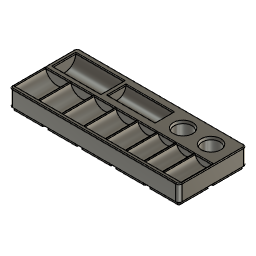
HarborFreightSocketHolder_LargeImperial (Autodesk Fusion 360 design; units mm, degrees)
Autodesk Fusion 360 part; units mm, degrees
sketch "Sketch1" plane through (0, 0, 0) normal (0, 0, 1) x (1, 0, 0) in component "Blank Storage"
  line L0 (0, 42) -> (42, 42)
  line L1 (42, 42) -> (42, 0)
  line L2 (42, 0) -> (0, 0)
  line L3 (0, 0) -> (0, 42)
  line L4 (0, 42) -> (42, 0) construction
  line L5 (42, 21) -> (0, 21) construction
  line L6 (42, 14.5) -> (0, 14.5)
  line L7 (42, 27.5) -> (0, 27.5)
  line L8 (27.5, 42) -> (27.5, 0)
  line L9 (14.5, 42) -> (14.5, 0)
  line L10 (14.5, 14.5) -> (0, 0) construction
  circle A0 centre (8, 8) radius 1.5
  circle A1 centre (34, 8) radius 1.5
  circle A2 centre (34, 34) radius 1.5
  circle A3 centre (8, 34) radius 1.5
  circle A4 centre (8, 8) radius 3.25
  circle A5 centre (34, 8) radius 3.25
  circle A6 centre (34, 34) radius 3.25
  circle A7 centre (8, 34) radius 3.25
  point P0 (21, 21)
  dimension "d1" = 42
  dimension "d2" = 42
  dimension "d65" = 13
  dimension "d67" = 90
  dimension "d69" = 3
  dimension "d71" = 360
  dimension "d80" = 6.5
  dimension "d85" = 8
  constraint horizontal L0
  constraint perpendicular L0 L1
  constraint parallel L0 L2
  constraint parallel L1 L3
  constraint coincident L2.end L3.start
  constraint midpoint L1 L5.start
  constraint midpoint L3 L5.end
  constraint coincident L1 L6.start
  constraint coincident L3 L6.end
  constraint perpendicular L3 L6
  constraint symmetric L5 L6.start L7.start
  constraint symmetric L5 L6.end L7.end
  constraint midpoint L4 P0
  constraint coincident L9 L10.start
  constraint coincident L6 L10.start
  constraint concentric A0 A4
  constraint coincident L10 A0.centre
  measures "d1" distance of L1.end L2.end
  measures "d2" distance of L0.end L1.end
  measures "d65" distance of L6 L7
  measures "d69" diameter of A0
  measures "d80" diameter of A4
  measures "d85" distance of L2 A0.centre
extrude "Extrude1" add sketch "Sketch1" along normal blind 5 contours L0 L3 L7 L9 | L0 L7 L8 L9 | L3 L6 L7 L9 | L0 L1 L7 L8 | L6 L7 L8 L9 | L2 L3 L6 L9 | L1 L6 L7 L8 | L2 L6 L8 L9 | L1 L2 L6 L8 | A0 | A1 | A2 | A3 | A4 | A5 | A6 | A7 makes body 1 in component "Blank Storage"
ref_plane "WorkPlane1" through (21, 21, 2.5) normal (0, -1, 0) x (1, 0, 0) in component "Blank Storage"
sketch "Sketch2" plane through (0, 21, 0) normal (0, -1, 0) x (1, 0, 0) in component "Blank Storage"
  line L0 (42, 0) -> (0, 0)
  line L1 (0, 0) -> (0, 5)
  line L2 (3.2, 0) -> (2.4, 0.8)
  line L3 (3.2, 0) -> (0, 0) construction
  line L4 (2.4, 0.8) -> (2.4, 2.6)
  line L5 (2.4, 2.6) -> (0, 5)
  line L6 (0, 5) -> (-5.1222, 5)
  line L7 (-5.1222, 5) -> (-5.1222, -0.0937)
  line L8 (-5.1222, -0.0937) -> (0, 0)
  dimension "d39" = 45
  dimension "d40" = 45
  dimension "d41" = 0.8
  dimension "d43" = 5
  dimension "d112" = 2.4
  constraint horizontal L3
  constraint coincident L0 L2.start
  constraint perpendicular L0 L4
  constraint coincident L1 L5.end
  constraint coincident L0.end L1.start
  constraint coincident L1.end L5.end
  constraint perpendicular L1 L6
  constraint perpendicular L6 L7
  measures "d39" angle of L2 L3
  measures "d40" angle of L4 L5
  measures "d41" distance of L2.end L3
  measures "d43" distance of L3 L1.end
  measures "d112" horizontal distance of L0.end L2.end
sketch "Sketch3" plane through (0, 0, 0) normal (0, 0, -1) x (1, 0, 0)
  line L0 (42, 0) -> (0, 0)
  line L1 (0, 0) -> (0, -42)
  line L2 (0, -42) -> (42, -42)
  line L3 (42, -42) -> (42, 0)
  arc A0 (4, 0) -> (0, -4) centre (4, -4) ccw
  line L4 (0, -42) -> (42, 0) construction
  arc A1 (0, -38) -> (4, -42) centre (4, -38) ccw
  arc A2 (38, -42) -> (42, -38) centre (38, -38) ccw
  arc A3 (42, -4) -> (38, 0) centre (38, -4) ccw
  line L5 (0, -4) -> (0, -38)
  line L6 (4, -42) -> (38, -42)
  line L7 (42, -38) -> (42, -4)
  line L8 (38, 0) -> (4, 0)
  point P0 (21, -21)
  dimension "d37" = 360
  constraint coincident L1.end L2.start
  constraint coincident L0.start L3.end
  constraint midpoint L4 P0
sweep "Sweep1" cut profiles "Sketch2" path "Sketch3" along L8 A0 L5 A1 L6 A2 L7 A3 section 1 bodies 1 in component "Blank Storage"
extrude "Extrude3" [suppressed] in component "Blank Storage"
draft "Draft1" [suppressed] in component "Blank Storage"
extrude "Extrude4" cut sketch "Sketch1" along normal up to surface (5 mm away) contours A0 | A1 | A2 | A3 bodies 1 in component "Blank Storage"
extrude "Extrude5" cut sketch "Sketch1" along normal blind 2.4 contours A4 | A5 | A6 | A7 bodies 1 in component "Blank Storage"
chamfer "Chamfer1" distance 1.75 angle 45 4 edges at (33.4576, 6.6015, 2.4) (35.3985, 33.4576, 2.4) (8.5424, 35.3985, 2.4) (6.6015, 8.5424, 2.4) on bodies 1 in component "Blank Storage"
pattern_linear "R-Pattern1" count 5 spacing 42 along (1, 0, 0) count 2 spacing 42 along (0, 1, 0) of bodies 1 makes body 2 at (66.9668, 17.0068, 5) makes body 3 at (24.9668, 59.0068, 5) makes body 4 at (66.9668, 59.0068, 5) makes body 5 at (108.9668, 17.0068, 5) makes body 6 at (108.9668, 59.0068, 5) makes body 7 at (150.9668, 17.0068, 5) makes body 8 at (192.9668, 17.0068, 5) makes body 9 at (150.9668, 59.0068, 5) makes body 10 at (192.9668, 59.0068, 5) in component "Blank Storage"
sketch "Sketch4" plane through (0, 0, 5) normal (0, 0, 1) x (-1, 0, 0) in component "Blank Storage"
  line L0 (-4, 0) -> (-206, 0)
  line L1 (-210, -4) -> (-210, -80)
  line L2 (-206, -84) -> (-4, -84)
  line L3 (0, -80) -> (0, -4)
  arc A0 (0, -4) -> (-4, 0) centre (-4, -4) ccw
  arc A1 (-206, 0) -> (-210, -4) centre (-206, -4) ccw
  arc A2 (-210, -80) -> (-206, -84) centre (-206, -80) ccw
  arc A3 (-4, -84) -> (0, -80) centre (-4, -80) ccw
  line L4 (-206, -83.75) -> (-4, -83.75)
  arc A4 (-4, -83.75) -> (-0.25, -80) centre (-4, -80) ccw
  line L5 (-0.25, -80) -> (-0.25, -4)
  arc A5 (-0.25, -4) -> (-4, -0.25) centre (-4, -4) ccw
  line L6 (-4, -0.25) -> (-206, -0.25)
  arc A6 (-206, -0.25) -> (-209.75, -4) centre (-206, -4) ccw
  line L7 (-209.75, -4) -> (-209.75, -80)
  arc A7 (-209.75, -80) -> (-206, -83.75) centre (-206, -80) ccw
  point P0 (-210, 0)
  point P1 (0, -84)
  dimension "d44" = 210
  dimension "d45" = 84
  dimension "d48" = 4
  dimension "d49" = 4
  dimension "d50" = 4
  dimension "d51" = 4
  dimension "d118" = -0.25
  constraint horizontal L0
  constraint vertical L1
  constraint horizontal L2
  constraint vertical L3
  constraint coincident origin L0
  constraint coincident origin L3
  constraint tangent L0 A0
  constraint tangent L3 A0
  constraint coincident P0 L0
  constraint coincident P0 L1
  constraint tangent L0 A1
  constraint tangent L1 A1
  constraint tangent L1 A2
  constraint tangent L2 A2
  constraint coincident P1 L2
  constraint coincident P1 L3
  constraint tangent L2 A3
  constraint tangent L3 A3
  measures "d44" distance of origin P0
  measures "d45" distance of origin P1
  measures "d48" radius of A0
  measures "d49" radius of A1
  measures "d50" radius of A2
  measures "d51" radius of A3
extrude "Extrude2" add sketch "Sketch4" along normal blind 20 contours L0 L1 L2 L3 A0 A1 A2 A3 | L4 A4 L5 A5 L6 A6 L7 A7 bodies 1 5 6 3 4 2 in component "Blank Storage"
ref_plane "WorkPlane2" through (105, 5, 15) normal (0, -1, 0) x (1, 0, 0)
sketch "Sketch7" plane through (105, 5, 15) normal (0, -1, 0) x (1, 0, 0)
  circle A0 centre (-88.4, 13) radius 15
  circle A1 centre (-58.4, 13) radius 14
  line L0 (-88.4, 13) -> (92.4, 13) construction
  circle A2 centre (-30.4, 13) radius 13
  circle A3 centre (22.5, 13) radius 11.9
  circle A4 centre (46.4, 13) radius 11
  circle A5 centre (69.4, 13) radius 11
  circle A6 centre (92.4, 13) radius 11
  circle A7 centre (-3.4, 13) radius 13
  line L1 (-101, 10) -> (101, 10)
  line L2 (-105, -10) -> (-105, 10)
  line L3 (105, -10) -> (105, 10)
  point P0 (-103.4, 13)
  point P1 (103.4, 13)
  point P2 (-73.4, 13)
  point P3 (-72.4, 13)
  point P4 (-44.4, 13)
  point P5 (-43.4, 13)
  point P6 (-17.4, 13)
  point P7 (-16.4, 13)
  point P8 (9.6, 13)
  point P9 (10.6, 13)
  point P10 (34.4, 13)
  point P11 (35.4, 13)
  point P12 (57.4, 13)
  point P13 (58.4, 13)
  point P14 (80.4, 13)
  point P15 (81.4, 13)
  dimension "d194" = 30
  dimension "d195" = 28
  dimension "d196" = 26
  dimension "d197" = 23.8
  dimension "d198" = 22
  dimension "d199" = 22
  dimension "d200" = 22
  dimension "d201" = 26
  dimension "d232" = 3
  dimension "d236" = 1
  dimension "d237" = 1
  dimension "d238" = 1
  dimension "d239" = 1
  dimension "d240" = 1
  dimension "d241" = 1
  dimension "d242" = 1
  dimension "d243" = 1.6
  dimension "d244" = 1.6
  constraint coincident A0.centre L0.start
  constraint horizontal L0
  constraint coincident A1.centre L0
  constraint coincident L0 A2.centre
  constraint coincident L0 A3.centre
  constraint coincident L0 A4.centre
  constraint coincident L0 A5.centre
  constraint coincident L0.end A6.centre
  constraint coincident L0 A7.centre
  constraint coincident A0 P0
  constraint coincident A6 P1
  constraint coincident L0 P1
  constraint coincident L0 P0
  constraint coincident A0 P2
  constraint coincident L0 P2
  constraint coincident A1 P3
  constraint coincident L0 P3
  constraint coincident A1 P4
  constraint coincident L0 P4
  constraint coincident A2 P5
  constraint coincident L0 P5
  constraint coincident A2 P6
  constraint coincident L0 P6
  constraint coincident A7 P7
  constraint coincident L0 P7
  constraint coincident A7 P8
  constraint coincident L0 P8
  constraint coincident A3 P9
  constraint coincident L0 P9
  constraint coincident A3 P10
  constraint coincident L0 P10
  constraint coincident A4 P11
  constraint coincident L0 P11
  constraint coincident A4 P12
  constraint coincident L0 P12
  constraint coincident A5 P13
  constraint coincident L0 P13
  constraint coincident A5 P14
  constraint coincident L0 P14
  constraint coincident A6 P15
  constraint coincident L0 P15
  measures "d194" diameter of A0
  measures "d195" diameter of A1
  measures "d196" diameter of A2
  measures "d197" diameter of A3
  measures "d198" diameter of A4
  measures "d199" diameter of A5
  measures "d200" diameter of A6
  measures "d201" diameter of A7
  measures "d232" distance of L0 L1
  measures "d236" distance of P2 P3
  measures "d237" distance of P4 P5
  measures "d238" distance of P6 P7
  measures "d239" distance of P8 P9
  measures "d240" distance of P10 P11
  measures "d241" distance of P12 P13
  measures "d242" distance of P14 P15
  measures "d243" horizontal distance of L2.end P0
  measures "d244" horizontal distance of L3.end P1
extrude "Extrude6" cut sketch "Sketch7" against normal blind 38 bodies 1 in component "Blank Storage"
ref_plane "WorkPlane3" through (5, 42, 15) normal (-1, 0, 0) x (0, -1, 0)
sketch "Sketch8" plane through (5, 42, 15) normal (-1, 0, 0) x (0, 1, 0)
  circle A0 centre (21.5, -10) radius 14
  line L0 (38, -10) -> (-38, -10)
  circle A1 centre (21.5, -10) radius 11
  point P0 (1, -10)
  point P1 (42, -10)
  dimension "d206" = 28
  dimension "d207" = 22
  dimension "d222" = 41
  dimension "d223" = 20.5
  constraint coincident A0.centre L0
  constraint concentric A0 A1
  measures "d206" diameter of A0
  measures "d207" diameter of A1
  measures "d222" distance of P0 P1
  measures "d223" distance of A0.centre P1
extrude "Extrude7" cut sketch "Sketch8" against normal blind 59 bodies 1 in component "Blank Storage"
extrude "Extrude8" cut sketch "Sketch8" against normal blind 58 from surface at -65 contours L0 A1 | L0 A1 bodies 1 in component "Blank Storage"
sketch "Sketch9" plane through (0, 0, 25) normal (0, 0, 1) x (-1, 0, 0)
  line L0 (-128, -52.5) -> (-70, -52.5)
  line L1 (-70, -52.5) -> (-70, -74.5)
  line L2 (-70, -74.5) -> (-128, -74.5)
  line L3 (-128, -74.5) -> (-128, -52.5)
  line L4 (-64, -49.5) -> (-5, -49.5)
  line L5 (-5, -49.5) -> (-5, -77.5)
  line L6 (-5, -77.5) -> (-64, -77.5)
  line L7 (-64, -77.5) -> (-64, -49.5)
  line L8 (-207.983, -43) -> (-207.983, -5)
  line L9 (-207.983, -5) -> (-186.817, -5)
  line L10 (-186.817, -43) -> (-207.983, -43)
  line L11 (-31.2969, -43) -> (-31.2969, -5)
  line L12 (-1.9031, -43) -> (-31.2969, -43)
  arc A0 (-4, -84) -> (0, -80) centre (-4, -80) ccw
  line L13 (0, -80) -> (0, -4)
  arc A1 (0, -4) -> (-4, 0) centre (-4, -4) ccw
  line L14 (-4, 0) -> (-206, 0)
  arc A2 (-206, 0) -> (-210, -4) centre (-206, -4) ccw
  line L15 (-210, -4) -> (-210, -80)
  arc A3 (-210, -80) -> (-206, -84) centre (-206, -80) ccw
  line L16 (-206, -84) -> (-4, -84)
  circle A4 centre (-151.6667, -63.5) radius 11
  circle A5 centre (-186.3333, -63.5) radius 11
  line L17 (-128, -63.5) -> (-210, -63.5) construction
  line L18 (-186.817, -5) -> (-186.817, -43)
  line L19 (-184.983, -43) -> (-184.983, -5)
  line L20 (-184.983, -5) -> (-163.817, -5)
  line L21 (-163.817, -5) -> (-163.817, -43)
  line L22 (-163.817, -43) -> (-184.983, -43)
  line L23 (-161.983, -43) -> (-161.983, -5)
  line L24 (-161.983, -5) -> (-140.817, -5)
  line L25 (-140.817, -5) -> (-140.817, -43)
  line L26 (-140.817, -43) -> (-161.983, -43)
  line L27 (-139.0156, -43) -> (-139.0156, -5)
  line L28 (-139.0156, -5) -> (-115.9844, -5)
  line L29 (-115.9844, -5) -> (-115.9844, -43)
  line L30 (-115.9844, -43) -> (-139.0156, -43)
  line L31 (-114.2491, -43) -> (-114.2491, -5)
  line L32 (-114.2491, -5) -> (-88.9509, -5)
  line L33 (-88.9509, -5) -> (-88.9509, -43)
  line L34 (-88.9509, -43) -> (-114.2491, -43)
  line L35 (-87.2491, -43) -> (-87.2491, -5)
  line L36 (-87.2491, -5) -> (-61.9509, -5)
  line L37 (-61.9509, -5) -> (-61.9509, -43)
  line L38 (-61.9509, -43) -> (-87.2491, -43)
  line L39 (-60.2748, -43) -> (-60.2748, -5)
  line L40 (-60.2748, -5) -> (-32.9252, -5)
  line L41 (-32.9252, -5) -> (-32.9252, -43)
  line L42 (-32.9252, -43) -> (-60.2748, -43)
  line L43 (-31.2969, -5) -> (-1.9031, -5)
  line L44 (-1.9031, -5) -> (-1.9031, -43)
  dimension "d213" = 22
  dimension "d214" = 22
  dimension "d215" = 82
  dimension "d218" = 23.6667
  dimension "d219" = 23.6667
  constraint midpoint L3 L17.start
  constraint coincident L15 L17.end
  constraint perpendicular L15 L17
  constraint coincident A5.centre L17
  constraint coincident A4.centre L17
  measures "d213" diameter of A4
  measures "d214" diameter of A5
  measures "d215" distance of L17.start L17.end
  measures "d218" distance of A4.centre L17.start
  measures "d219" distance of A5.centre L17.end
extrude "Extrude9" cut sketch "Sketch9" against normal blind 18 contours A4 | A5 bodies 1 in component "Blank Storage"
chamfer "Chamfer3" distance 1 distance2 3 2 edges at (196.5889, 59.5222, 25) (161.9223, 59.5222, 25) measured on face at (205.0645, 61.6202, 25) measured on face at (205.0645, 61.6202, 25) on bodies 1 in component "Blank Storage"
fillet "Fillet6" radius 1 48 edges at (32.9252, 24, 25) (31.2969, 24, 25) (60.2748, 24, 25) (61.9509, 24, 25) (87.2491, 24, 25) (88.9509, 24, 25) (114.2491, 24, 25) (115.9844, 24, 25) (139.0156, 24, 25) (140.817, 24, 25) (161.983, 24, 25) (163.817, 24, 25) (184.983, 24, 25) (186.817, 24, 25) (207.983, 24, 25) (16.6, 43, 25) (46.6, 43, 25) (74.6, 43, 25) (101.6, 43, 25) (127.5, 43, 25) (151.4, 43, 25) (174.4, 43, 25) (197.4, 43, 25) (197.4, 5, 25) (174.4, 5, 25) (151.4, 5, 25) (127.5, 5, 25) (101.6, 5, 25) (74.6, 5, 25) (46.6, 5, 25) (16.6, 5, 25) (1.9031, 24, 25) (105, 0, 25) (208.8284, 1.1716, 25) (210, 42, 25) (208.8284, 82.8284, 25) (105, 84, 25) (1.1716, 82.8284, 25) (0, 42, 25) (1.1716, 1.1716, 25) (34.5, 77.5, 25) (64, 63.5, 25) (5, 63.5, 25) (34.5, 49.5, 25) (99, 52.5, 25) (70, 63.5, 25) (99, 74.5, 25) (128, 63.5, 25) on bodies 1 in component "Blank Storage"
component "Blank Storage" placed x (1, 0, 0) y (0, 1, 0) z (0, 0, 1) at (0, 0, 0)
equation "d1 = slotDimension"
equation "d2 = slotDimension"
equation "d3 = nestingDepth"
equation "slotsWide = 5"
equation "slotsHigh = 1 / 2"
equation "slotsDeep = 2"
equation "slotDimension = 42 mm"
equation "nestingDepth = 5 mm"
equation "nestingRimWidth = 2.4 mm"
equation "nestingClearance = 0.25 mm"
equation "cornerFillet = 4 mm"
equation "d31 = slotsWide"
equation "d32 = slotsDeep"
equation "d33 = slotDimension"
equation "d34 = slotDimension"
equation "d38 = -slotDimension / 2"
equation "d43 = nestingDepth"
equation "d44 = slotDimension * slotsWide"
equation "d45 = slotDimension * slotsDeep"
equation "d48 = cornerFillet"
equation "d49 = cornerFillet"
equation "d50 = cornerFillet"
equation "d51 = cornerFillet"
equation "ledStripWidth = 13 mm"
equation "ledSlotHeight = 4 mm"
equation "d65 = ledStripWidth"
equation "screwTightDiameter = 3 mm"
equation "d69 = screwTightDiameter"
equation "d72 = ledSlotHeight"
equation "magnetDiameter = 6.5 mm"
equation "magnetThiccness = 2.4 mm"
equation "d80 = magnetDiameter"
equation "d81 = magnetThiccness"
equation "wallThiccness = 1.2 mm"
equation "d112 = nestingRimWidth"
equation "d138 = 126.00 mm"
equation "d139 = d138 / 6"
equation "d146 = d138 / 5"
equation "d151 = d138 / 4"
equation "d152 = d151"
equation "LabelHeight = 10 mm"
equation "d216 = d215 / 3"
equation "d218 = ( d215 - d213 - d214 ) / 3 + d213 / 2"
equation "d219 = d218"
equation "d223 = d222 / 2"
equation "d237 = d236"
equation "d238 = d236"
equation "d239 = d236"
equation "d240 = d236"
equation "d241 = d236"
equation "d242 = d236"
named bodies: "Body1 (1)"
